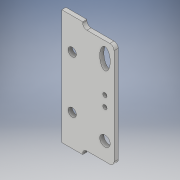
# Autodesk Inventor part: Radio Chip Plate
Saved by Autodesk Inventor 2019 (Build 230136000, 136)
## iProperties
Created: 2019-10-06
Part Number: Radio Chip Plate
Material: Generic
Document SubType Name: Modeling
Designer: robgr
Density: 1 g/cm^3
Appearance: Default
Author: robgr
Autodesk Inventor part; units mm, degrees
ref_plane "YZ Plane" through (0, 0, 0) normal (1, 0, 0) x (0, 1, 0)
ref_plane "XZ Plane" through (0, 0, 0) normal (0, 1, 0) x (-1, 0, 0)
ref_plane "XY Plane" through (0, 0, 0) normal (0, 0, 1) x (1, 0, 0)
sketch "Sketch1" plane through (0, 0, 0) normal (0, 0, 1) x (1, 0, 0)
  line L0 (0, 44.009) -> (10, 44.009)
  line L1 (0, -10.991) -> (0, 44.009)
  line L2 (10, 44.009) -> (10, 43.509)
  line L3 (25, 39.509) -> (25, -6.491)
  line L4 (23, 41.509) -> (12, 41.509)
  line L5 (23, -8.491) -> (12, -8.491)
  line L6 (0, -10.991) -> (10, -10.991)
  arc A0 (10, 43.509) -> (12, 41.509) centre (12, 43.509) ccw
  line L7 (10, -10.991) -> (10, -10.491)
  arc A1 (12, -8.491) -> (10, -10.491) centre (12, -10.491) ccw
  arc A2 (25, 39.509) -> (23, 41.509) centre (23, 39.509) ccw
  arc A3 (23, -8.491) -> (25, -6.491) centre (23, -6.491) ccw
  circle A4 centre (5, 29.009) radius 2
  circle A5 centre (5, 4.009) radius 2
  circle A6 centre (20.6584, 0) radius 2.5
  ellipse E0 centre (20.6584, 34.0813) end of major axis (20.6584, 29.0813) minor radius 2.508
  circle A7 centre (20.6584, 19.009) radius 1
  circle A8 centre (20.6584, 14.009) radius 1
  line L8 (25, 16.509) -> (0, 16.509)
  point P0 (0, 0)
  point P1 (25, 41.509)
  point P2 (25, -8.491)
  point P3 (10, -8.491)
  dimension "d11" = 5
  dimension "d1" = 55
  dimension "d3" = 50
  dimension "d6" = 2
  dimension "d7" = 2
  dimension "d8" = 2
  dimension "d9" = 4
  dimension "d10" = 5
  dimension "d12" = 2
  dimension "d13" = 2
  dimension "d23" = 4
  dimension "d24" = 25
  dimension "d26" = 12.5
  dimension "d27" = 5
  dimension "d28" = 5
  constraints: 18 end point, 9 centre point, 8 point on circle, 8 point on line, 8 tangent, 3 perpendicular, 2 midpoint, 2 vertical, 1 equal radius, 1 horizontal, 2 other
  measures "d1" distance of L1.start L0.start
  measures "d3" distance of point (25, 41.509) point (25, -8.491)
  measures "d6" radius of A0
  measures "d7" radius of A1
  measures "d8" radius of A2
  measures "d9" diameter of A4
  measures "d10" diameter of A6
  measures "d12" diameter of A7
  measures "d13" diameter of A8
  measures "d23" diameter of A5
  measures "d24" distance of A5.centre A4.centre
  measures "d26" distance from line of L8 A5.centre
  measures "d27" distance from line of L1 A5.centre
  measures "d28" distance from line of L1 A4.centre
extrude "Extrusion1" add sketch "Sketch1" along normal blind 2
body "Solid1"
